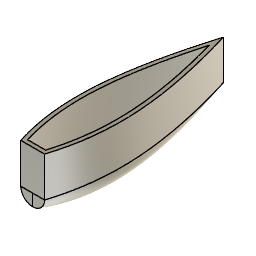
test lod 4 (Autodesk Fusion 360 design; units mm, degrees)
part number: 2025-10-20-20-40-49-444
Autodesk Fusion 360 part; units mm, degrees
sketch "Sketch1" plane through (0, 0, 0) normal (0, 0, 1) x (1, 0, 0)
  line L0 (0, 0) -> (0, 480) construction
  line L1 (32.5, 261.3008) -> (-32.5, 261.3008)
  line L2 (-32.5, 261.3008) -> (-32.5, 105.3008)
  line L3 (-32.5, 105.3008) -> (32.5, 105.3008)
  line L4 (32.5, 105.3008) -> (32.5, 261.3008)
  line L5 (32.5, 183.3008) -> (-32.5, 183.3008) construction
  line L6 (0, 261.3008) -> (0, 105.3008) construction
  line L7 (-32.5, 105.3008, 0) -> (-32.5, 105.3008, -100)
  line L8 (-32.5, 105.3008, -100) -> (-32.5, 261.3008, -100)
  line L9 (-32.5, 261.3008, -100) -> (-32.5, 261.3008, 0)
  line L10 (-32.5, 261.3008) -> (-32.5, 105.3008)
  line L11 (-32.5, 105.3008, -100) -> (32.5, 105.3008, -100)
  line L12 (32.5, 105.3008, -100) -> (32.5, 105.3008, 0)
  line L13 (32.5, 105.3008) -> (-32.5, 105.3008)
  line L14 (-32.5, 105.3008, 0) -> (-32.5, 105.3008, -100)
  line L15 (32.5, 261.3008, 0) -> (32.5, 261.3008, -100)
  line L16 (32.5, 261.3008, -100) -> (32.5, 105.3008, -100)
  line L17 (32.5, 105.3008, -100) -> (32.5, 105.3008, 0)
  line L18 (32.5, 105.3008) -> (32.5, 261.3008)
  line L19 (32.5, 261.3008, 0) -> (32.5, 261.3008, -100)
  line L20 (32.5, 261.3008, -100) -> (-32.5, 261.3008, -100)
  line L21 (-32.5, 261.3008, -100) -> (-32.5, 261.3008, 0)
  line L22 (-32.5, 261.3008) -> (32.5, 261.3008)
  line L23 (-30, 0) -> (30, 0)
  line L24 (30, 0, 0) -> (30, 0, -100)
  line L25 (30, 0, -100) -> (-30, 0, -100)
  line L26 (-30, 0, -100) -> (-30, 0, 0)
  spline S0 degree 5 poles (30, 0) (32.4439, 7.6481) (37.052, 23.1237) (43.1249, 46.8753) (49.5162, 79.6379) (54.4829, 122.5293) (56.2074, 167.4998) (54.5077, 214.6659) (49.4269, 264.0003) (41.2201, 315.3391) (30.1826, 368.4931) (19.3003, 412.3323) (10.0619, 445.9021) (3.4324, 468.5837) (0, 480) knots 0 0 0 0 0 0 0.1 0.2 0.3 0.4 0.5 0.6 0.7 0.8 0.9 1 1 1 1 1 1
  line L27 (0, 480) -> (0, 440)
  line L28 (-22.6417, 10) -> (22.6417, 10)
  spline S1 degree 3 poles (22.6417, 10) (30.821, 36.9415) (36.9376, 65.242) (40.7676, 95.0278) (44.3762, 123.0907) (45.9174, 152.4988) (45.166, 183.4437) (44.4078, 214.6749) (41.3031, 247.49) (36.1016, 281.7315) (30.0133, 321.8117) (21.11, 363.7988) (9.9316, 407.289) (6.7998, 419.4737) (3.488, 431.7773) (0, 444.1965) knots 0.018479 0.018479 0.018479 0.018479 0.232261 0.232261 0.232261 0.433677 0.433677 0.433677 0.636956 0.636956 0.636956 0.874898 0.874898 0.874898 0.941562 0.941562 0.941562 0.941562
  spline S2 degree 5 poles (-30, 0) (-32.4439, 7.6481) (-37.052, 23.1237) (-43.1249, 46.8753) (-49.5162, 79.6379) (-54.4829, 122.5293) (-56.2074, 167.4998) (-54.5077, 214.6659) (-49.4269, 264.0003) (-41.2201, 315.3391) (-30.1826, 368.4931) (-19.3003, 412.3323) (-10.0619, 445.9021) (-3.4324, 468.5837) (0, 480) knots 0 0 0 0 0 0 0.1 0.2 0.3 0.4 0.5 0.6 0.7 0.8 0.9 1 1 1 1 1 1
  line L29 (15.9224, -44.0549) -> (44.0776, 44.0549)
  line L30 (15.955, 426.9333) -> (-15.955, 533.0667)
  line L31 (-15.9224, -44.0549) -> (-44.0776, 44.0549)
  line L32 (-15.955, 426.9333) -> (15.955, 533.0667)
  spline S3 degree 3 poles (-22.6417, 10) (-30.821, 36.9415) (-36.9376, 65.242) (-40.7676, 95.0278) (-44.3762, 123.0907) (-45.9174, 152.4988) (-45.166, 183.4437) (-44.4078, 214.6749) (-41.3031, 247.49) (-36.1016, 281.7315) (-30.0133, 321.8117) (-21.11, 363.7988) (-9.9316, 407.289) (-6.7998, 419.4737) (-3.488, 431.7773) (0, 444.1965) knots 0.018479 0.018479 0.018479 0.018479 0.232261 0.232261 0.232261 0.433677 0.433677 0.433677 0.636956 0.636956 0.636956 0.874898 0.874898 0.874898 0.941562 0.941562 0.941562 0.941562
  line L33 (22.6417, 10) -> (-22.6417, 10)
  spline S4 degree 5 poles (-30, 0, -100) (-32.4439, 7.6481, -100) (-37.052, 23.1237, -100) (-43.1249, 46.8753, -100) (-49.5162, 79.6379, -100) (-54.4829, 122.5293, -100) (-56.2074, 167.4998, -100) (-54.5077, 214.6659, -100) (-49.4269, 264.0003, -100) (-41.2201, 315.3391, -100) (-30.1826, 368.4931, -100) (-19.3003, 412.3323, -100) (-10.0619, 445.9021, -100) (-3.4324, 468.5837, -100) (0, 480, -100) knots 0 0 0 0 0 0 0.1 0.2 0.3 0.4 0.5 0.6 0.7 0.8 0.9 1 1 1 1 1 1
  line L34 (-15.9224, -44.0549, -100) -> (-44.0776, 44.0549, -100)
  line L35 (-15.955, 426.9333, -100) -> (15.955, 533.0667, -100)
  spline S5 degree 3 poles (-22.6417, 10, -100) (-30.821, 36.9415, -100) (-36.9376, 65.242, -100) (-40.7676, 95.0278, -100) (-44.3762, 123.0907, -100) (-45.9174, 152.4988, -100) (-45.166, 183.4437, -100) (-44.4078, 214.6749, -100) (-41.3031, 247.49, -100) (-36.1016, 281.7315, -100) (-30.0133, 321.8117, -100) (-21.11, 363.7988, -100) (-9.9316, 407.289, -100) (-6.7998, 419.4737, -100) (-3.488, 431.7773, -100) (0, 444.1965, -100) knots 0.01847946 0.01847946 0.01847946 0.01847946 0.23226094 0.23226094 0.23226094 0.43367666 0.43367666 0.43367666 0.63695616 0.63695616 0.63695616 0.87489772 0.87489772 0.87489772 0.94156205 0.94156205 0.94156205 0.94156205
  spline S6 degree 3 poles (22.6417, 10, -100) (30.821, 36.9415, -100) (36.9376, 65.242, -100) (40.7676, 95.0278, -100) (44.3762, 123.0907, -100) (45.9174, 152.4988, -100) (45.166, 183.4437, -100) (44.4078, 214.6749, -100) (41.3031, 247.49, -100) (36.1016, 281.7315, -100) (30.0133, 321.8117, -100) (21.11, 363.7988, -100) (9.9316, 407.289, -100) (6.7998, 419.4737, -100) (3.488, 431.7773, -100) (0, 444.1965, -100) knots 0.01847946 0.01847946 0.01847946 0.01847946 0.23226094 0.23226094 0.23226094 0.43367666 0.43367666 0.43367666 0.63695616 0.63695616 0.63695616 0.87489772 0.87489772 0.87489772 0.94156205 0.94156205 0.94156205 0.94156205
  spline S7 degree 5 poles (30, 0, -100) (32.4439, 7.6481, -100) (37.052, 23.1237, -100) (43.1249, 46.8753, -100) (49.5162, 79.6379, -100) (54.4829, 122.5293, -100) (56.2074, 167.4998, -100) (54.5077, 214.6659, -100) (49.4269, 264.0003, -100) (41.2201, 315.3391, -100) (30.1826, 368.4931, -100) (19.3003, 412.3323, -100) (10.0619, 445.9021, -100) (3.4324, 468.5837, -100) (0, 480, -100) knots 0 0 0 0 0 0 0.1 0.2 0.3 0.4 0.5 0.6 0.7 0.8 0.9 1 1 1 1 1 1
  line L36 (15.9224, -44.0549, -100) -> (44.0776, 44.0549, -100)
  line L37 (15.955, 426.9333, -100) -> (-15.955, 533.0667, -100)
  line L38 (0, 480, -100) -> (0, 440, -100)
  line L39 (22.6417, 10, -100) -> (-22.6417, 10, -100)
  line L40 (-30, 0, -100) -> (30, 0, -100)
  line L41 (0, 480, 0) -> (0, 480, -140)
  line L42 (0, 480, -100) -> (0, 480, 0)
  line L43 (0, 0, 0) -> (0, 0, -140)
  line L44 (0, 480, -140) -> (0, 440, -140)
  line L45 (0, 480, -100) -> (0, 440, -140)
  line L46 (0, 480, -100) -> (11.1078, 441.5732, -100)
  line L47 (11.1078, 441.5732, -100) -> (0, 440, -140)
  line L48 (11.1078, 441.5732, -100) -> (21.366, 402.911, -100)
  line L49 (21.366, 402.911, -100) -> (0, 400, -140)
  line L50 (0, 400, -140) -> (0, 440, -140)
  line L51 (11.1078, 441.5732, -100) -> (0, 400, -140)
  line L52 (0, 400, -140) -> (0, 360, -140)
  line L53 (0, 360, -140) -> (0, 320, -140)
  line L54 (0, 320, -140) -> (0, 280, -140)
  line L55 (0, 280, -140) -> (0, 240, -140)
  line L56 (0, 240, -140) -> (0, 200, -140)
  line L57 (0, 200, -140) -> (0, 160, -140)
  line L58 (0, 160, -140) -> (0, 120, -140)
  line L59 (0, 120, -140) -> (0, 80, -140)
  line L60 (0, 80, -140) -> (0, 40, -140)
  line L61 (0, 40, -140) -> (0, 0, -140)
  line L62 (21.366, 402.911, -100) -> (0, 360, -140)
  line L63 (21.366, 402.911, -100) -> (30.5246, 363.9736, -100)
  line L64 (30.5246, 363.9736, -100) -> (0, 360, -140)
  line L65 (30.5246, 363.9736, -100) -> (38.8122, 324.8416, -100)
  line L66 (38.8122, 324.8416, -100) -> (0, 320, -140)
  line L67 (30.5246, 363.9736, -100) -> (0, 320, -140)
  line L68 (38.8122, 324.8416, -100) -> (45.6519, 285.4307, -100)
  line L69 (45.6519, 285.4307, -100) -> (0, 280, -140)
  line L70 (38.8122, 324.8416, -100) -> (0, 280, -140)
  line L71 (45.6519, 285.4307, -100) -> (50.9064, 245.7773, -100)
  line L72 (50.9064, 245.7773, -100) -> (0, 240, -140)
  line L73 (45.6519, 285.4307, -100) -> (0, 240, -140)
  line L74 (50.9064, 245.7773, -100) -> (54.2547, 205.9177, -100)
  line L75 (54.2547, 205.9177, -100) -> (0, 200, -140)
  line L76 (50.9064, 245.7773, -100) -> (0, 200, -140)
  line L77 (54.2547, 205.9177, -100) -> (55.3494, 165.9327, -100)
  line L78 (55.3494, 165.9327, -100) -> (0, 160, -140)
  line L79 (54.2547, 205.9177, -100) -> (0, 160, -140)
  line L80 (55.3494, 165.9327, -100) -> (0, 120, -140)
  line L81 (55.3494, 165.9327, -100) -> (53.8857, 125.9594, -100)
  line L82 (53.8857, 125.9594, -100) -> (0, 120, -140)
  line L83 (53.8857, 125.9594, -100) -> (49.6595, 86.1833, -100)
  line L84 (49.6595, 86.1833, -100) -> (0, 80, -140)
  line L85 (53.8857, 125.9594, -100) -> (0, 80, -140)
  line L86 (49.6595, 86.1833, -100) -> (42.5574, 46.8189, -100)
  line L87 (42.5574, 46.8189, -100) -> (0, 40, -140)
  line L88 (42.5574, 46.8189, -100) -> (0, 0, -140)
  line L89 (49.6595, 86.1833, -100) -> (0, 40, -140)
  line L90 (30, 0, -100) -> (0, 0, -140)
  line L91 (42.5574, 46.8189, -100) -> (30, 0, -100)
  line L92 (0, 0, -100) -> (0, 10, -100)
  point P0 (0, 183.3008)
  point P1 (55, 189.3876)
  point P2 (-55, 189.3876)
  point P3 (55, 189.3876)
  point P4 (-55, 189.3876)
  dimension "d1" = 480
  dimension "d5" = 65
  dimension "d6" = 156
  dimension "d9" = 100
  dimension "d12" = 100
  dimension "d19" = 30
  dimension "d20" = 55
  dimension "d23" = 140
  dimension "d24" = 100
  dimension "d27" = 140
  dimension "d31" = 40
  dimension "d33" = 40
  dimension "d34" = 40
  dimension "d35" = 40
  dimension "d36" = 40
  dimension "d37" = 40
  dimension "d38" = 40
  dimension "d39" = 40
  dimension "d40" = 40
  dimension "d41" = 40
  dimension "d42" = 40
  dimension "d43" = 40
  dimension "d44" = 40
  dimension "d45" = 40
  dimension "d46" = 40
  dimension "d47" = 40
  dimension "d48" = 40
  dimension "d49" = 40
  dimension "d50" = 40
  dimension "d51" = 40
  dimension "d52" = 40
  dimension "d53" = 40
  dimension "d54" = 40
  constraint vertical L0
  constraint coincident L0.start origin
  constraint horizontal L1
  constraint vertical L2
  constraint horizontal L3
  constraint vertical L4
  constraint midpoint L4 L5.start
  constraint midpoint L2 L5.end
  constraint midpoint L1 L6.start
  constraint midpoint L3 L6.end
  constraint midpoint L5 P0
  constraint coincident L0 P0
  constraint vertical L10
  constraint horizontal L13
  constraint vertical L18
  constraint horizontal L22
  constraint horizontal L23
  constraint coincident L0 L27.end
  constraint coincident L0 S1.end
  constraint midpoint L23.end L29
  constraint midpoint L0.end L30
  constraint symmetric S0.end L0 L27.start
  constraint symmetric L0 L23.end L23.start
  constraint symmetric L0 P3 P4
  constraint symmetric L0 S1.end S3.end
  constraint symmetric L0 L28.end L28.start
  constraint symmetric L0 S1 S3
  constraint symmetric L0 L29.start L31.start
  constraint symmetric L0 L29.end L31.end
  constraint symmetric L0 L30.start L32.start
  constraint symmetric L0 L30.end L32.end
  measures "d1" distance of L0.start L0.end
  measures "d5" distance of L1.start L1.end
  measures "d6" distance of L1.start L3.end
  measures "d9" distance of L2.end L3.start
  measures "d12" distance of L23.start S2.start
  measures "d19" distance of L0.start L23.end
  measures "d20" horizontal distance of L0.start P3
  measures "d23" distance of L0.end S0.end
  measures "d27" distance of L0.start origin
  measures "d31" distance of L0.end L27.end
extrude "Extrude2" add sketch "Sketch1" against normal blind 100 contours L23 S0 S2 makes body 1
revolve "Revolve1" add sketch "Sketch1" angle 90 about axis through (0, 0, -100) along (0, -1, 0) separate body contours L25 S4 S5 L38 L39 L40 L92 in plane through (0, 0, -100) normal (0, 0, 1) makes body 2
mirror "Mirror1" about plane through (0, 0, -100) normal (1, 0, 0) of "Revolve1" makes body 3
equation "d12 = d24"
equation "d27 = d23"
equation "q = 40 mm"
equation "d31 = q"
equation "d33 = q"
equation "d34 = q"
equation "d35 = q"
equation "d36 = q"
equation "d37 = q"
equation "d38 = q"
equation "d39 = q"
equation "d40 = q"
equation "d41 = q"
equation "d42 = q"
equation "d43 = q"
equation "d44 = q"
equation "d45 = q"
equation "d46 = q"
equation "d47 = q"
equation "d48 = q"
equation "d49 = q"
equation "d50 = q"
equation "d51 = q"
equation "d52 = q"
equation "d53 = q"
equation "d54 = q"
